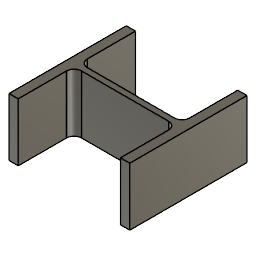
H-208×202×10×16 (Autodesk Fusion 360 design; units mm, degrees)
Autodesk Fusion 360 part; units mm, degrees
sketch "スケッチ1" plane through (0, 0, 0) normal (0, 0, 1) x (1, 0, 0)
  line L0 (0, 101) -> (0, -101)
  line L1 (208, -101) -> (208, 101)
  line L2 (29, -5) -> (179, -5)
  line L3 (16, -101) -> (16, -18)
  line L4 (0, -101) -> (16, -101)
  arc A0 (29, -5) -> (16, -18) centre (29, -18) ccw
  line L5 (192, -18) -> (192, -101)
  line L6 (192, -101) -> (208, -101)
  arc A1 (192, -18) -> (179, -5) centre (179, -18) ccw
  line L7 (179, 5) -> (29, 5)
  line L8 (16, 18) -> (16, 101)
  arc A2 (16, 18) -> (29, 5) centre (29, 18) ccw
  line L9 (16, 101) -> (0, 101)
  line L10 (192, 101) -> (192, 18)
  arc A3 (179, 5) -> (192, 18) centre (179, 18) ccw
  line L11 (208, 101) -> (192, 101)
extrude "押し出し1" add sketch "スケッチ1" along normal blind 100
